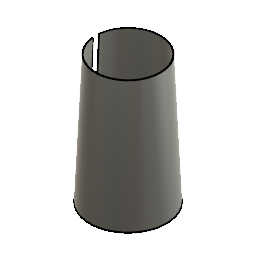
Cable Holder v1 (Autodesk Fusion 360 design; units mm, degrees)
Autodesk Fusion 360 part; units mm, degrees
note: some values were not read from the file. Chosen so that the rebuilt part matches the saved one: which pieces of a blend or face edit are solid. Set by a fixed rule: which sketch regions a step uses.
sketch "Sketch1" plane through (0, 0, 0) normal (0, 0, 1) x (1, 0, 0)
  line L0 (0, 0) -> (-45, 0)
  line L1 (-45, 0) -> (-45, 1)
  line L2 (-45, 1) -> (0, 1)
  line L3 (0, 1) -> (0, 0)
  line L4 (-35, 200) -> (-36, 200)
  line L5 (-36, 200) -> (-45, 1)
  line L6 (-45, 1) -> (-44, 1)
  line L7 (-44, 1) -> (-35, 200)
  dimension "d2" = 45
  dimension "d3" = 1
  dimension "d5" = 1
  constraint horizontal L0
  constraint vertical L1
  constraint horizontal L2
  constraint vertical L3
  constraint coincident L0.start L3.end
  constraint horizontal L4
  constraint coincident L2 L6.end
  measures "d2" distance of L0.start L0.end
  measures "d3" distance of L0.start L2.end
  measures "d5" distance of L4.start L4.end
revolve "Revolve1" add sketch "Sketch1" angle 360 about axis through (0, 1, 0) along (0, -1, 0)
sketch "Sketch2" plane through (0, 200, 0) normal (0, 1, 0) x (-1, 0, 0)
  circle A0 centre (0, 0) radius 36
  circle A1 centre (0, 0) radius 35
  line L0 (35, 0) -> (59, 0)
  line L1 (59, 0) -> (59, -3.5)
  line L2 (59, -3.5) -> (29, -3.5)
  line L3 (29, -3.5) -> (29, 3.5)
  line L4 (29, 3.5) -> (59, 3.5)
  line L5 (59, 3.5) -> (59, -3.5)
  point P0 (35, 0)
  dimension "d7" = 3.5
  dimension "d8" = 7
  constraint coincident P0 L0.start
  constraint horizontal L0
  constraint perpendicular L0 L1
  constraint horizontal L2
  constraint vertical L3
  constraint horizontal L4
  constraint vertical L5
  measures "d7" distance of L0.end L1.end
  measures "d8" distance of L1.end L4.end
extrude "Extrude1" cut sketch "Sketch2" against normal blind 199 contours A0 A1 L0 L4 | A0 L0 L1 L2 L5 | A0 A1 L0 L2 | A0 L0 L4 L5 | A1 L2 L3 L4 picked at (31, 0)
move_face "OffsetFaces1" offset -50 1 faces at (-35.1904, 200, 5.2542)
